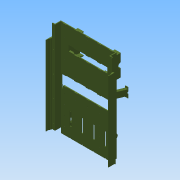
# Autodesk Inventor part: 载板上盖
Saved by Autodesk Inventor 2015 (Build 190159000, 159)
## iProperties
Created: 2017-05-12
Part Number: 载板上盖
Material: 常规
Document SubType Name: Modeling
Designer: Administrator
Density: 1 g/cm^3
Appearance: 橄榄绿
Author: Administrator
Autodesk Inventor part; units mm, degrees
ref_plane "YZ Plane" through (0, 0, 0) normal (1, 0, 0) x (0, 1, 0)
ref_plane "XZ Plane" through (0, 0, 0) normal (0, 1, 0) x (-1, 0, 0)
ref_plane "XY Plane" through (0, 0, 0) normal (0, 0, 1) x (1, 0, 0)
sketch "草图1" plane through (0, 0, 0) normal (0, 0, 1) x (1, 0, 0)
  line L0 (325, 8) -> (325, 0)
  line L1 (325, 0) -> (-325, 0)
  line L2 (-325, 0) -> (-325, 8)
  line L3 (-325, 0) -> (-320, 0)
  line L4 (-320, 0) -> (-320, -52.5)
  line L5 (-320, -52.5) -> (-325, -52.5)
  line L6 (-325, -52.5) -> (-325, 0)
  line L7 (-315, -12.5) -> (-310, -12.5)
  line L8 (-310, -12.5) -> (-310, 0)
  line L9 (325, 0) -> (320, 0)
  line L10 (320, 0) -> (320, -52.5)
  line L11 (320, -52.5) -> (325, -52.5)
  line L12 (325, -52.5) -> (325, 0)
  line L13 (310, 0) -> (310, -12.5)
  line L14 (310, -12.5) -> (315, -12.5)
  line L15 (315, -12.5) -> (315, -22.5)
  line L16 (315, -22.5) -> (320, -27.5)
  line L17 (-315, -12.5) -> (-315, -22.5)
  line L18 (-315, -22.5) -> (-320, -27.5)
  line L19 (-288, 0) -> (-280, 0)
  line L20 (-280, 0) -> (-280, 60)
  line L21 (-280, 60) -> (-288, 60)
  line L22 (-288, 60) -> (-288, 0)
  line L23 (288, 0) -> (280, 0)
  line L24 (280, 0) -> (280, 60)
  line L25 (280, 60) -> (288, 60)
  line L26 (288, 60) -> (288, 0)
  line L27 (-288, 60) -> (288, 60)
  line L28 (288, 60) -> (288, 68)
  line L29 (288, 68) -> (-288, 68)
  line L30 (-288, 68) -> (-288, 60)
  line L31 (-325, 8) -> (-280, 8)
  line L32 (280, 8) -> (325, 8)
  point P0 (0, 0)
  point P1 (0, 0)
  dimension "d0" = 650
  dimension "d1" = 8
  dimension "d2" = 5
  dimension "d3" = 52.5
  dimension "d4" = 12.5
  dimension "d5" = 5
  dimension "d8" = 5
  dimension "d9" = 12.5
  dimension "d10" = 5
  dimension "d11" = 10
  dimension "d12" = 5
  dimension "d14" = 45
  dimension "d15" = 10
  dimension "d16" = 5
  dimension "d17" = 135
  dimension "d18" = 10
  dimension "d19" = 8
  dimension "d20" = 30
  dimension "d21" = 60
  dimension "d22" = 8
  dimension "d23" = 30
  dimension "d24" = 60
  dimension "d25" = 8
  dimension "d26" = 8
  constraints: 66 end point, 14 parallel, 10 perpendicular, 8 point on line, 7 horizontal, 2 vertical, 1 coincident, 1 collinear, 1 midpoint
  measures "d0" distance of L0.end L1.end
  measures "d1" distance of L0.start L0.end
  measures "d2" distance of L4.end L5.end
  measures "d3" distance of L5.end L1.end
  measures "d4" distance of L7.end L8.end
  measures "d5" distance of L7.start L7.end
  measures "d8" distance of L11.end L10.end
  measures "d9" distance of L13.start L13.end
  measures "d10" distance of L13.end L14.end
  measures "d11" distance of L14.end L15.end
  measures "d12" distance from line of L10 L15.end
  measures "d14" angle of L10 L16
  measures "d15" distance of L7.start L17.end
  measures "d16" distance between parallel lines of L4 L17
  measures "d17" angle of L4 L18
  measures "d18" distance between parallel lines of L4 L8
  measures "d19" distance of L21.end L20.end
  measures "d20" distance between parallel lines of L8 L20
  measures "d21" distance of L21.end L19.start
  measures "d22" distance of L24.end L25.end
  measures "d23" distance between parallel lines of L13 L24
  measures "d24" distance of L25.end L23.start
  measures "d25" distance between parallel lines of L27 L29
  measures "d26" distance between parallel lines of L1 L31
extrude "拉伸1" add sketch "草图1" along normal blind 900 contours L0 L1 L26 L32 | L12 L11 L10 L1 | L32 L24 L25 L26 | L26 L1 L24 L32 | L10 L16 L15 L14 L13 L1 | L25 L27 L21 L30 L29 L28 | L20 L31 L22 L21 | L1 L22 L31 L20 | L1 L2 L31 L22 | L8 L7 L17 L18 L4 L1 | L4 L5 L6 L1
sketch "草图2" plane through (-325, -52.5, 0) normal (-1, 0, 0) x (0, 0, 1)
  line L0 (767.5, 60.5) -> (900, 60.5)
  line L1 (900, 60.5) -> (900, 0)
  line L2 (900, 0) -> (767.5, 0)
  line L3 (767.5, 0) -> (767.5, 60.5)
  line L4 (0, 60.5) -> (900, 60.5) projected
  point P0 (0, 52.5)
  dimension "d29" = 132.5
  constraints: 8 end point, 2 parallel, 1 coincident, 1 collinear, 1 horizontal, 1 perpendicular
  measures "d29" distance of L1.end L2.end
extrude "拉伸2" cut sketch "草图2" against normal blind 15
sketch "草图3" plane through (325, -52.5, 0) normal (1, 0, 0) x (0, 0, -1)
  line L0 (-900, 0) -> (-767.5, 0)
  line L1 (-767.5, 0) -> (-767.5, 60.5)
  line L2 (-767.5, 60.5) -> (-900, 60.5)
  line L3 (-900, 60.5) -> (-900, 0)
  line L4 (0, 60.5) -> (-900, 60.5) projected
  point P0 (0, 52.5)
  dimension "d32" = 132.5
  constraints: 8 end point, 2 parallel, 1 collinear, 1 horizontal, 1 perpendicular
  measures "d32" distance of L0.start L0.end
extrude "拉伸3" cut sketch "草图3" against normal blind 15
sketch "草图4" plane through (-325, 8, 0) normal (0, 1, 0) x (1, 0, 0)
  circle A0 centre (26, -10) radius 4
  line L0 (0, 0) -> (0, -767.5) projected
  line L1 (37, 0) -> (0, 0) projected
  circle A1 centre (624, -10) radius 4
  line L2 (650, 0) -> (650, -767.5) projected
  line L3 (650, 0) -> (613, 0) projected
  point P0 (325, 0)
  dimension "d35" = 8
  dimension "d36" = 26
  dimension "d37" = 10
  dimension "d38" = 8
  dimension "d39" = 26
  dimension "d40" = 10
  constraints: 2 centre point
  measures "d35" diameter of A0
  measures "d36" distance from line of L0 A0.centre
  measures "d37" distance from line of L1 A0.centre
  measures "d38" diameter of A1
  measures "d39" distance from line of L2 A1.centre
  measures "d40" distance from line of L3 A1.centre
extrude "拉伸4" cut sketch "草图4" against normal blind 8
pattern_linear "矩形阵列1" count 5 spacing 220 along (0, 0, 1) of "拉伸4"
sketch "草图5" plane through (0, 0, 0) normal (0, 0, -1) x (-1, 0, 0)
  line L0 (-288, 8) -> (-325, 8)
  line L1 (-325, 8) -> (-288, 8) projected
  line L2 (-325, 8) -> (-325, -52.5)
  line L3 (-325, -52.5) -> (-320.7269, -52.5)
  line L4 (-320.7269, -52.5) -> (-320, -52.5)
  line L5 (-320, -27.5) -> (-320, -52.5) projected
  line L6 (-320, -52.5) -> (-320, -27.5)
  line L7 (-320, -27.5) -> (-315, -22.5)
  line L8 (-315, -22.5) -> (-320, -27.5) projected
  line L9 (-315, -22.5) -> (-315, -12.5)
  line L10 (-315, -12.5) -> (-310, -12.5)
  line L11 (-310, -12.5) -> (-315, -12.5) projected
  line L12 (-310, -12.5) -> (-310, 0)
  line L13 (-310, 0) -> (-280, 0)
  line L14 (-280, 0) -> (-280, 60)
  line L15 (-280, 60) -> (280, 60)
  line L16 (280, 60) -> (280, 0)
  line L17 (280, 0) -> (310, 0)
  line L18 (310, 0) -> (280, 0) projected
  line L19 (310, 0) -> (310, -12.5)
  line L20 (310, -12.5) -> (315, -12.5)
  line L21 (315, -12.5) -> (310, -12.5) projected
  line L22 (315, -12.5) -> (315, -22.5)
  line L23 (315, -22.5) -> (315, -12.5) projected
  line L24 (315, -22.5) -> (320, -27.5)
  line L25 (320, -27.5) -> (315, -22.5) projected
  line L26 (320, -27.5) -> (320, -52.5)
  line L27 (320, -52.5) -> (325, -52.5)
  line L28 (325, -52.5) -> (325, 8)
  line L29 (325, 8) -> (288, 8)
  line L30 (288, 8) -> (288, 68)
  line L31 (288, 68) -> (-288, 68)
  line L32 (-288, 68) -> (-288, 8)
  point P0 (0, 0)
  constraints: 50 end point, 15 perpendicular, 8 collinear, 2 parallel, 1 point on line
extrude "拉伸5" add sketch "草图5" along normal blind 50
sketch "草图6" plane through (-288, 68, 900) normal (0, 1, 0) x (1, 0, 0)
  line L0 (89, 172) -> (487, 172)
  line L1 (487, 172) -> (487, 228)
  line L2 (487, 228) -> (89, 228)
  line L3 (89, 228) -> (89, 172)
  line L4 (288, 228) -> (288, 172)
  line L5 (89, 200) -> (487, 200)
  line L6 (576, 0) -> (0, 0) projected
  line L7 (613, 950) -> (613, 132.5) projected
  point P0 (288, 900)
  dimension "d48" = 398
  dimension "d49" = 56
  dimension "d50" = 200
  dimension "d51" = 325
  constraints: 12 end point, 4 midpoint, 2 parallel, 1 horizontal, 1 perpendicular
  measures "d48" distance of L2.end L1.end
  measures "d49" distance of L2.end L0.start
  measures "d50" distance between parallel lines of L6 L5
  measures "d51" distance between parallel lines of L7 L4
extrude "拉伸6" cut sketch "草图6" against normal through all
sketch "草图7" plane through (-288, 68, 900) normal (0, 1, 0) x (1, 0, 0)
  line L0 (526, 460) -> (15, 460)
  line L1 (15, 460) -> (15, 560)
  line L2 (15, 560) -> (526, 560)
  line L3 (526, 560) -> (526, 460)
  line L4 (576, 0) -> (0, 0) projected
  line L5 (0, 950) -> (0, 0) projected
  line L6 (576, 950) -> (576, 0) projected
  point P0 (288, 900)
  dimension "d54" = 460
  dimension "d55" = 560
  dimension "d56" = 15
  dimension "d57" = 50
  constraints: 8 end point, 2 parallel, 1 horizontal, 1 perpendicular
  measures "d54" distance between parallel lines of L4 L0
  measures "d55" distance between parallel lines of L4 L2
  measures "d56" distance between parallel lines of L5 L1
  measures "d57" distance between parallel lines of L6 L3
extrude "拉伸7" cut sketch "草图7" against normal blind 8
sketch "草图8" plane through (-288, 68, 900) normal (0, 1, 0) x (1, 0, 0)
  line L0 (115.5, 892) -> (100.5, 892)
  line L1 (100.5, 892) -> (100.5, 755)
  line L2 (100.5, 755) -> (115.5, 755)
  line L3 (115.5, 755) -> (115.5, 892)
  line L4 (576, 0) -> (0, 0) projected
  line L5 (0, 950) -> (0, 0) projected
  point P0 (288, 900)
  dimension "d60" = 15
  dimension "d61" = 755
  dimension "d62" = 892
  dimension "d63" = 100.5
  constraints: 8 end point, 2 parallel, 1 horizontal, 1 perpendicular
  measures "d60" distance of L1.end L2.end
  measures "d61" distance between parallel lines of L4 L2
  measures "d62" distance between parallel lines of L4 L0
  measures "d63" distance between parallel lines of L5 L1
extrude "拉伸8" cut sketch "草图8" against normal blind 8
pattern_linear "矩形阵列2" count 4 spacing 120 along (1, 0, 0) of "拉伸8"
sketch "草图9" plane through (0, 0, 900) normal (0, 0, 1) x (1, 0, 0)
  line L0 (-273, 60) -> (238, 60) projected
  line L1 (-225, 60) -> (-220, 55)
  line L2 (-220, 55) -> (-260, 55)
  line L3 (-260, 55) -> (-255, 60)
  line L4 (-280, 0) -> (-280, 60) projected
  point P0 (0, 0)
  dimension "d69" = 20
  dimension "d70" = 40
  dimension "d71" = 30
  dimension "d72" = 25
  dimension "d73" = 5
  constraints: 6 end point, 2 point on line, 1 parallel
  measures "d69" distance from line of L4 L2.end
  measures "d70" distance of L2.end L1.end
  measures "d71" distance of L1.start L3.end
  measures "d72" distance from line of L4 L3.end
  measures "d73" distance between parallel lines of L0 L2
extrude "拉伸9" add sketch "草图9" against normal blind 950
pattern_linear "矩形阵列3" count 5 spacing 120 along (1, 0, 0) of "拉伸9"
sketch "草图10" plane through (-288, 68, 900) normal (0, 1, 0) x (1, 0, 0)
  line L0 (526, 560) -> (15, 560)
  line L1 (15, 560) -> (15, 460)
  line L2 (15, 460) -> (526, 460)
  line L3 (487, 228) -> (89, 228)
  line L4 (89, 172) -> (487, 172)
  line L5 (513, 460) -> (513, 560) projected
  line L6 (526, 460) -> (15, 460) projected
  line L7 (15, 560) -> (526, 560) projected
  line L8 (15, 460) -> (15, 560) projected
  line L9 (89, 228) -> (89, 172)
  line L10 (487, 172) -> (89, 172) projected
  line L11 (89, 228) -> (487, 228) projected
  line L12 (487, 228) -> (487, 172)
  line L13 (526, 460) -> (526, 560)
  line L14 (513, 460) -> (526, 460) projected
  point P0 (288, 900)
  constraints: 16 end point, 6 point on line, 5 collinear, 2 horizontal, 2 parallel, 2 perpendicular, 2 vertical
extrude "拉伸10" cut sketch "草图10" against normal blind 13
sketch "草图11" plane through (-260, 55, 900) normal (0, -1, 0) x (1, 0, 0)
  circle A0 centre (20, -25) radius 2.5
  line L0 (0, 0) -> (40, 0) projected
  line L1 (0, 0) -> (0, -460) projected
  point P0 (260, -900)
  dimension "d81" = 5
  dimension "d82" = 25
  dimension "d83" = 20
  constraints: 1 centre point
  measures "d81" diameter of A0
  measures "d82" distance from line of L0 A0.centre
  measures "d83" distance from line of L1 A0.centre
extrude "拉伸11" cut sketch "草图11" against normal blind 13
thread "螺纹1" size "M5x0.8" class "6H" standard "ANSI Metric M Profile" full length
pattern_linear "矩形阵列4" count 5 spacing 100 along (0, 0, -1) of "拉伸11" skipped copies 3
sketch "草图12" plane through (-260, 55, 340) normal (0, -1, 0) x (1, 0, 0)
  circle A0 centre (20, -365) radius 2.5
  line L0 (40, -390) -> (0, -390) projected
  point P0 (260, -340)
  dimension "d91" = 5
  dimension "d92" = 25
  dimension "d93" = 20
  constraints: 1 centre point
  measures "d91" diameter of A0
  measures "d92" distance from line of L0 A0.centre
  measures "d93" horizontal distance of L0.start A0.centre
extrude "拉伸12" cut sketch "草图12" against normal blind 13
thread "螺纹2" size "M5x0.8" class "6H" standard "ANSI Metric M Profile" full length
pattern_linear "矩形阵列5" count 4 spacing 100 along (0, 0, 1) of "拉伸12"
pattern_linear "矩形阵列6" count 5 spacing 120 along (1, 0, 0) of "拉伸11", "矩形阵列4", "拉伸12", "矩形阵列5"
sketch "草图13" plane through (-288, 68, 900) normal (0, 1, 0) x (1, 0, 0)
  line L0 (523, 710) -> (40, 710)
  line L1 (40, 710) -> (40, 690)
  line L2 (40, 690) -> (523, 690)
  line L3 (523, 690) -> (523, 710)
  line L4 (0, 950) -> (0, 0) projected
  line L5 (576, 0) -> (0, 0) projected
  point P0 (288, 900)
  dimension "d104" = 483
  dimension "d105" = 40
  dimension "d106" = 20
  dimension "d107" = 690
  constraints: 8 end point, 2 parallel, 1 horizontal, 1 perpendicular
  measures "d104" distance of L2.end L1.end
  measures "d105" distance between parallel lines of L4 L1
  measures "d106" distance of L0.end L1.end
  measures "d107" distance between parallel lines of L5 L2
extrude "拉伸13" add sketch "草图13" along normal blind 22
fillet "圆角1" radius 10 2 edges at (-6.5, 90, 190) (-6.5, 90, 210)
sketch "草图14" plane through (-248, 68, 190) normal (-1, 0, 0) x (0, 0, 1)
  circle A0 centre (10, 12) radius 5
  arc A1 (20, 12) -> (0, 12) centre (10, 12) ccw projected
  point P0 (-190, -68)
  dimension "d111" = 10
  constraints: 1 centre point, 1 concentric
  measures "d111" diameter of A0
extrude "拉伸14" cut sketch "草图14" against normal through all
sketch "草图15" plane through (-288, 68, 900) normal (0, 1, 0) x (1, 0, 0)
  line L0 (40, 710) -> (523, 710) projected
  line L1 (523, 690) -> (40, 690) projected
  line L2 (100, 710) -> (181, 710)
  line L3 (181, 710) -> (181, 690)
  line L4 (181, 690) -> (100, 690)
  line L5 (100, 690) -> (100, 710)
  line L6 (241, 690) -> (322, 690)
  line L7 (322, 690) -> (322, 710)
  line L8 (322, 710) -> (241, 710)
  line L9 (241, 710) -> (241, 690)
  line L10 (382, 690) -> (463, 690)
  line L11 (463, 690) -> (463, 710)
  line L12 (463, 710) -> (382, 710)
  line L13 (382, 710) -> (382, 690)
  line L14 (40, 690) -> (40, 710) projected
  line L15 (523, 710) -> (523, 690) projected
  point P0 (288, 900)
  dimension "d114" = 81
  dimension "d115" = 81
  dimension "d116" = 81
  dimension "d117" = 60
  dimension "d118" = 60
  dimension "d119" = 60
  constraints: 24 end point, 6 parallel, 6 point on line, 3 horizontal, 3 perpendicular
  measures "d114" distance of L3.end L4.end
  measures "d115" distance of L8.end L7.end
  measures "d116" distance of L12.end L11.end
  measures "d117" distance between parallel lines of L14 L5
  measures "d118" distance from line of L10.end L15
  measures "d119" distance between parallel lines of L7 L13
extrude "拉伸15" cut sketch "草图15" along normal through all contours L0 L3 L1 L5 | L0 L7 L1 L9 | L0 L11 L1 L13
ref_plane "工作平面1" through (-248, 8, 900) normal (-1, 0, 0) x (0, 0, 1)
sketch "草图16" plane through (-248, 8, 900) normal (-1, 0, 0) x (0, 0, 1)
  line L0 (-950, 60) -> (0, 60) projected
  line L1 (-450, 60) -> (-502.3989, 235.379)
  line L2 (-390.5103, 60) -> (-450, 60)
  line L3 (-390.5103, 60) -> (-442.9091, 235.379)
  line L4 (-502.3989, 235.379) -> (-442.9091, 235.379)
  line L5 (0, 60) -> (0, 0) projected
  line L6 (-522.654, 235.379) -> (-422.654, 235.379)
  line L7 (-422.654, 235.379) -> (-422.654, 230.379)
  line L8 (-422.654, 230.379) -> (-522.654, 230.379)
  line L9 (-522.654, 230.379) -> (-522.654, 235.379)
  arc A0 (-483.154, 235.379) -> (-462.154, 235.379) centre (-472.654, 235.379) ccw
  line L10 (-441.4153, 230.379) -> (-442.9091, 235.379)
  line L11 (-422.654, 235.379) -> (-422.654, 230.379)
  line L12 (-502.3989, 235.379) -> (-522.654, 235.379)
  line L13 (-522.654, 230.379) -> (-500.905, 230.379)
  line L14 (-502.3989, 235.379) -> (-500.905, 230.379)
  line L15 (-500.905, 230.379) -> (-522.654, 230.379)
  line L16 (-522.654, 230.379) -> (-522.654, 235.379)
  line L17 (-522.654, 235.379) -> (-502.3989, 235.379)
  point P0 (-900, -8)
  dimension "d123" = 57
  dimension "d124" = 175.379
  dimension "d125" = 450
  dimension "d126" = 472.654
  dimension "d127" = 100
  dimension "d128" = 5
  dimension "d129" = 10.5
  constraints: 32 end point, 8 point on line, 6 collinear, 3 parallel, 2 coincident, 2 horizontal, 2 midpoint, 2 perpendicular, 2 point on circle, 1 centre point, 1 vertical
  measures "d123" distance between parallel lines of L3 L1
  measures "d124" distance between parallel lines of L0 L4
  measures "d125" distance from line of L5 point (-450, 60)
  measures "d126" distance from line of point (-472.654, 235.379) L5
  measures "d127" distance of L7.end L8.end
  measures "d128" distance of L6.end L7.end
  measures "d129" radius of A0
extrude "拉伸16" add sketch "草图16" against normal blind 30 contours L1 L8 A0 L3 L0 | L8 L9 L6 L1 | L1 L4 A0 L8 | L8 A0 L4 L3 | L3 L6 L7 L8
pattern_linear "矩形阵列7" count 2 spacing 453 along (1, 0, 0) of "拉伸16"
sketch "草图17" plane through (-218, 8, 900) normal (1, 0, 0) x (0, 0, -1)
  circle A0 centre (472.654, 235.379) radius 18.5
  arc A1 (462.154, 235.379) -> (483.154, 235.379) centre (472.654, 235.379) ccw projected
  point P0 (900, -8)
  dimension "d135" = 37
  constraints: 1 centre point, 1 concentric
  measures "d135" diameter of A0
extrude "拉伸17" cut sketch "草图17" against normal blind 9
sketch "草图18" plane through (-227, 8, 900) normal (1, 0, 0) x (0, 0, -1)
  circle A0 centre (472.654, 235.379) radius 14
  arc A1 (462.154, 235.379) -> (483.154, 235.379) centre (472.654, 235.379) ccw projected
  point P0 (900, -8)
  dimension "d138" = 28
  constraints: 1 centre point, 1 concentric
  measures "d138" diameter of A0
extrude "拉伸18" cut sketch "草图18" against normal blind 5
sketch "草图19" plane through (205, 243.379, 437.846) normal (-1, 0, 0) x (0, 0, 1)
  circle A0 centre (-10.5, 0) radius 18.5
  arc A1 (-21, 0) -> (0, 0) centre (-10.5, 0) ccw projected
  point P0 (-437.846, -243.379)
  dimension "d141" = 37
  constraints: 1 centre point, 1 concentric
  measures "d141" diameter of A0
extrude "拉伸19" cut sketch "草图19" against normal blind 9
sketch "草图20" plane through (214, 243.379, 437.846) normal (-1, 0, 0) x (0, 0, 1)
  circle A0 centre (-10.5, 0) radius 14
  arc A1 (-21, 0) -> (0, 0) centre (-10.5, 0) ccw projected
  point P0 (-437.846, -243.379)
  dimension "d144" = 28
  constraints: 1 centre point, 1 concentric
  measures "d144" diameter of A0
extrude "拉伸20" cut sketch "草图20" against normal blind 5
fillet "圆角2" radius 4 8 edges at (-233, 238.379, 458.5847) (-233, 238.379, 399.095) (-233, 68, 509.4897) (-233, 68, 450) (220, 68, 450) (220, 68, 509.4897) (220, 238.379, 458.5847) (220, 238.379, 399.095)
sketch "草图21" plane through (-248, 243.379, 477.346) normal (0, 1, 0) x (1, 0, 0)
  circle A0 centre (7, 7) radius 2.5
  circle A1 centre (23, 7) radius 2.5
  circle A2 centre (7, 93) radius 2.5
  circle A3 centre (23, 93) radius 2.5
  line L0 (30, 100) -> (30, 68.5) projected
  line L1 (0, 100) -> (30, 100) projected
  line L2 (0, 100) -> (0, 81.2306) projected
  line L3 (30, 31.5) -> (30, 0) projected
  line L4 (0, 0) -> (30, 0) projected
  line L5 (0, 0) -> (0, 39.5) projected
  point P0 (248, 477.346)
  dimension "d148" = 5
  dimension "d149" = 5
  dimension "d150" = 5
  dimension "d151" = 5
  dimension "d152" = 7
  dimension "d153" = 7
  dimension "d154" = 7
  dimension "d155" = 7
  dimension "d156" = 7
  dimension "d157" = 7
  dimension "d158" = 7
  dimension "d159" = 7
  constraints: 4 centre point
  measures "d148" diameter of A0
  measures "d149" diameter of A1
  measures "d150" diameter of A2
  measures "d151" diameter of A3
  measures "d152" distance from line of L0 A3.centre
  measures "d153" distance from line of A3.centre L1
  measures "d154" distance from line of L1 A2.centre
  measures "d155" distance from line of L2 A2.centre
  measures "d156" distance from line of L3 A1.centre
  measures "d157" distance from line of L4 A1.centre
  measures "d158" distance from line of L4 A0.centre
  measures "d159" distance from line of L5 A0.centre
extrude "拉伸21" cut sketch "草图21" against normal blind 5
pattern_linear "矩形阵列8" count 2 spacing 453 along (1, 0, 0) of "拉伸21"
sketch "草图22" plane through (-248, 8, 900) normal (-1, 0, 0) x (0, 0, 1)
  circle A0 centre (-800, 99.5) radius 25
  line L0 (-821.6506, 112) -> (-851.6728, 60)
  line L1 (-892, 60) -> (-755, 60) projected
  line L2 (-950, 60) -> (0, 60) projected
  line L3 (-748.3272, 60) -> (-778.3494, 112)
  line L4 (-851.6728, 60) -> (-748.3272, 60)
  line L5 (0, 60) -> (0, 0) projected
  point P0 (-900, -8)
  dimension "d165" = 50
  dimension "d166" = 60
  dimension "d167" = 39.5
  dimension "d168" = 800
  constraints: 6 end point, 2 point on circle, 2 point on line, 2 tangent, 1 centre point, 1 collinear, 1 equal length
  measures "d165" diameter of A0
  measures "d166" angle of L2 L3
  measures "d167" distance from line of L1 A0.centre
  measures "d168" distance from line of L5 A0.centre
extrude "拉伸22" add sketch "草图22" against normal blind 18
pattern_linear "矩形阵列9" count 2 spacing 465 along (1, 0, 0) of "拉伸22"
sketch "草图23" plane through (-248, 8, 900) normal (-1, 0, 0) x (0, 0, 1)
  circle A0 centre (-800, 99.5) radius 25
  arc A1 (-778.3494, 112) -> (-821.6506, 112) centre (-800, 99.5) ccw projected
  line L0 (-892, 60) -> (-755, 60) projected
  line L1 (-825, 60) -> (-825, 106.1987)
  line L2 (-851.6728, 60) -> (-821.6506, 112) projected
  line L3 (-775, 60) -> (-775, 106.1987)
  line L4 (-778.3494, 112) -> (-748.3272, 60) projected
  line L5 (-825, 106.1987) -> (-821.6506, 112)
  arc A2 (-778.3494, 112) -> (-821.6506, 112) centre (-800, 99.5) ccw projected
  line L6 (-775, 106.1987) -> (-778.3494, 112)
  line L7 (-825, 60) -> (-775, 60)
  point P0 (-900, -8)
  dimension "d174" = 50
  constraints: 10 end point, 4 point on line, 4 tangent, 1 centre point, 1 collinear, 1 concentric, 1 horizontal, 1 parallel, 1 vertical
  measures "d174" diameter of A0
extrude "拉伸23" cut sketch "草图23" against normal blind 5 contours A0 | L3 L0 L1 A0 | A0 L4 L3 | L1 L2 A0
sketch "草图24" plane through (-243, 8, 900) normal (-1, 0, 0) x (0, 0, 1)
  circle A0 centre (-800, 99.5) radius 16
  arc A1 (-778.3494, 112) -> (-821.6506, 112) centre (-800, 99.5) ccw projected
  point P0 (-900, -8)
  dimension "d177" = 32
  constraints: 1 centre point, 1 concentric
  measures "d177" diameter of A0
extrude "拉伸24" cut sketch "草图24" against normal blind 13
sketch "草图25" plane through (217, 107.5, 100) normal (-1, 0, 0) x (0, 0, 1)
  circle A0 centre (0, 0) radius 16
  arc A1 (21.6506, 12.5) -> (-21.6506, 12.5) centre (0, 0) ccw projected
  point P0 (-100, -107.5)
  dimension "d180" = 32
  constraints: 1 centre point, 1 concentric
  measures "d180" diameter of A0
extrude "拉伸25" cut sketch "草图25" against normal blind 9
sketch "草图26" plane through (226, 107.5, 100) normal (-1, 0, 0) x (0, 0, 1)
  circle A0 centre (0, 0) radius 12
  circle A1 centre (0, 0) radius 16 projected
  point P0 (-100, -107.5)
  dimension "d183" = 24
  constraints: 1 centre point, 1 concentric
  measures "d183" diameter of A0
extrude "拉伸26" cut sketch "草图26" against normal blind 3 contours A0
sketch "草图27" plane through (229, 107.5, 100) normal (-1, 0, 0) x (0, 0, 1)
  circle A0 centre (0, 0) radius 7.5
  circle A1 centre (0, 0) radius 12 projected
  point P0 (-100, -107.5)
  dimension "d186" = 15
  constraints: 1 centre point, 1 concentric
  measures "d186" diameter of A0
extrude "拉伸27" cut sketch "草图27" against normal through all contours A0
sketch "草图28" plane through (-243, 8, 900) normal (-1, 0, 0) x (0, 0, 1)
  circle A0 centre (-815, 70) radius 2
  circle A1 centre (-785, 70) radius 2
  circle A2 centre (-785, 113.4732) radius 2
  circle A3 centre (-815, 113.4732) radius 2
  line L0 (-775, 106.1987) -> (-775, 60) projected
  line L1 (-950, 60) -> (0, 60) projected
  line L2 (-825, 60) -> (-825, 106.1987) projected
  arc A4 (-785, 113.4732) -> (-815, 113.4732) centre (-800, 99.5) ccw
  arc A5 (-778.3494, 112) -> (-821.6506, 112) centre (-800, 99.5) ccw projected
  point P0 (-900, -8)
  dimension "d189" = 4
  dimension "d190" = 4
  dimension "d191" = 4
  dimension "d192" = 4
  dimension "d193" = 10
  dimension "d194" = 10
  dimension "d195" = 10
  dimension "d196" = 10
  dimension "d197" = 20.5
  dimension "d198" = 10
  dimension "d199" = 10
  constraints: 5 centre point, 2 point on circle, 1 concentric
  measures "d189" diameter of A0
  measures "d190" diameter of A1
  measures "d191" diameter of A2
  measures "d192" diameter of A3
  measures "d193" distance from line of A1.centre L0
  measures "d194" distance from line of L1 A1.centre
  measures "d195" distance from line of L1 A0.centre
  measures "d196" distance from line of L2 A0.centre
  measures "d197" radius of A4
  measures "d198" distance from line of L0 A2.centre
  measures "d199" distance from line of L2 A3.centre
extrude "拉伸28" cut sketch "草图28" against normal blind 13
sketch "草图29" plane through (-288, 68, 900) normal (0, 1, 0) x (1, 0, 0)
  line L0 (66, 310) -> (89, 310)
  line L1 (89, 310) -> (89, 90)
  line L2 (89, 90) -> (66, 90)
  line L3 (66, 90) -> (66, 310)
  line L4 (576, 0) -> (0, 0) projected
  line L5 (0, 950) -> (0, 0) projected
  line L6 (487, 310) -> (510, 310)
  line L7 (510, 310) -> (510, 90)
  line L8 (510, 90) -> (487, 90)
  line L9 (487, 90) -> (487, 310)
  line L10 (576, 950) -> (576, 0) projected
  point P0 (288, 900)
  dimension "d202" = 23
  dimension "d203" = 90
  dimension "d204" = 66
  dimension "d205" = 220
  dimension "d206" = 23
  dimension "d207" = 90
  dimension "d208" = 66
  dimension "d209" = 220
  constraints: 16 end point, 4 parallel, 2 horizontal, 2 perpendicular
  measures "d202" distance of L1.end L2.end
  measures "d203" distance between parallel lines of L4 L2
  measures "d204" distance between parallel lines of L5 L3
  measures "d205" distance of L0.end L1.end
  measures "d206" distance of L7.end L8.end
  measures "d207" distance between parallel lines of L4 L8
  measures "d208" distance between parallel lines of L10 L7
  measures "d209" distance of L8.end L6.start
extrude "拉伸29" add sketch "草图29" along normal blind 109.5
sketch "草图30" plane through (-222, 68, 590) normal (-1, 0, 0) x (0, 0, 1)
  circle A0 centre (110, 109.5) radius 26
  line L0 (0, 109.5) -> (220, 109.5) projected
  point P0 (-590, -68)
  point P1 (110, 109.5)
  dimension "d212" = 52
  constraints: 1 centre point, 1 coincident, 1 midpoint
  measures "d212" diameter of A0
extrude "拉伸30" cut sketch "草图30" against normal through all
sketch "草图31" plane through (-222, 68, 590) normal (-1, 0, 0) x (0, 0, 1)
  circle A0 centre (84.3674, 83.8674) radius 2.5
  circle A1 centre (135.6326, 83.8674) radius 2.5
  arc A2 (84.3674, 83.8674) -> (135.6326, 83.8674) centre (110, 109.5) ccw
  arc A3 (84, 109.5) -> (136, 109.5) centre (110, 109.5) ccw projected
  line L0 (135.6326, 83.8674) -> (110, 109.5)
  line L1 (110, 109.5) -> (84.3674, 83.8674)
  line L2 (136, 109.5) -> (220, 109.5) projected
  point P0 (-590, -68)
  dimension "d215" = 5
  dimension "d216" = 5
  dimension "d217" = 36.25
  dimension "d218" = 45
  constraints: 4 end point, 3 centre point, 2 point on circle, 1 concentric, 1 perpendicular
  measures "d215" diameter of A0
  measures "d216" diameter of A1
  measures "d217" radius of A2
  measures "d218" angle of L2 L0
extrude "拉伸31" cut sketch "草图31" against normal through all contours A0 A2 L1 | L1 A2 A0 | A2 L0 A1 | A1 L0 A2
thread "螺纹3" size "M5x0.8" class "6H" standard "ANSI Metric M Profile" full length
thread "螺纹4" size "M5x0.8" class "6H" standard "ANSI Metric M Profile" full length
thread "螺纹5" size "M5x0.8" class "6H" standard "ANSI Metric M Profile" full length
thread "螺纹6" size "M5x0.8" class "6H" standard "ANSI Metric M Profile" full length
sketch "草图32" plane through (199, 60, 672) normal (-1, 0, 0) x (0, 0, 1)
  arc A0 (2, 117.5) -> (54, 117.5) centre (28, 117.5) ccw projected
  line L0 (138, 117.5) -> (54, 117.5) projected
  line L1 (131, 117.5) -> (138, 117.5)
  line L2 (138, 117.5) -> (138, 8)
  line L3 (138, 8) -> (138, 117.5) projected
  line L4 (138, 8) -> (-82, 8)
  line L5 (-82, 8) -> (-82, 117.5)
  line L6 (-82, 8) -> (-82, 117.5) projected
  line L7 (-82, 117.5) -> (-75, 117.5)
  line L8 (2, 117.5) -> (-82, 117.5) projected
  line L9 (0, 18.3789) -> (0, 8)
  line L10 (138, 8) -> (-82, 8) projected
  line L11 (56, 18.3789) -> (56, 8)
  arc A1 (56, 18.3789) -> (131, 117.5) centre (28, 117.5) ccw
  arc A2 (-75, 117.5) -> (0, 18.3789) centre (28, 117.5) ccw
  arc A3 (2, 117.5) -> (54, 117.5) centre (28, 117.5) ccw projected
  point P0 (-672, -60)
  dimension "d230" = 56
  dimension "d231" = 103
  dimension "d232" = 103
  constraints: 14 end point, 4 point on circle, 4 point on line, 3 equal length, 2 centre point, 1 concentric, 1 horizontal, 1 parallel, 1 perpendicular, 1 vertical
  measures "d230" distance between parallel lines of L11 L9
  measures "d231" radius of A2
  measures "d232" radius of A1
extrude "拉伸32" add sketch "草图32" along normal blind 38 contours A2 L9 L4 L5 L7 | L0 L2 L4 L11 A1
pattern_linear "矩形阵列10" count 2 spacing 360 along (-1, 0, 0) of "拉伸32"
sketch "草图33" plane through (-288, 177.5, 900) normal (0, 1, 0) x (1, 0, 0)
  circle A0 centre (498.5, 255) radius 4
  circle A1 centre (498.5, 145) radius 4
  circle A2 centre (77.5, 255) radius 4
  circle A3 centre (77.5, 145) radius 4
  line L0 (510, 90) -> (449, 90) projected
  line L1 (510, 226) -> (510, 310) projected
  line L2 (510, 90) -> (510, 174) projected
  line L3 (66, 90) -> (127, 90) projected
  line L4 (89, 226) -> (89, 303) projected
  line L5 (89, 97) -> (89, 174) projected
  point P0 (288, 900)
  dimension "d238" = 8
  dimension "d239" = 8
  dimension "d240" = 8
  dimension "d241" = 8
  dimension "d242" = 110
  dimension "d243" = 55
  dimension "d244" = 11.5
  dimension "d245" = 11.5
  dimension "d246" = 110
  dimension "d247" = 55
  dimension "d248" = 11.5
  dimension "d249" = 11.5
  constraints: 4 centre point
  measures "d238" diameter of A0
  measures "d239" diameter of A1
  measures "d240" diameter of A2
  measures "d241" diameter of A3
  measures "d242" distance of A1.centre A0.centre
  measures "d243" distance from line of L0 A1.centre
  measures "d244" distance from line of L1 A0.centre
  measures "d245" distance from line of L2 A1.centre
  measures "d246" distance of A3.centre A2.centre
  measures "d247" distance from line of L3 A3.centre
  measures "d248" distance from line of L4 A2.centre
  measures "d249" distance from line of L5 A3.centre
extrude "拉伸33" cut sketch "草图33" against normal blind 22
thread "螺纹7" size "M8x1.25" class "6H" standard "ANSI Metric M Profile" full length
thread "螺纹8" size "M8x1.25" class "6H" standard "ANSI Metric M Profile" full length
thread "螺纹9" size "M8x1.25" class "6H" standard "ANSI Metric M Profile" full length
thread "螺纹10" size "M8x1.25" class "6H" standard "ANSI Metric M Profile" full length
sketch "草图34" plane through (0, 0, -50) normal (0, 0, -1) x (-1, 0, 0)
  line L0 (288, 68) -> (-288, 68) projected
  line L1 (-280, 68) -> (280, 68)
  line L2 (280, 68) -> (280, 60)
  line L3 (280, 60) -> (-280, 60)
  line L4 (-280, 60) -> (-280, 68)
  line L5 (-280, 0) -> (-280, 60) projected
  line L6 (-280, 60) -> (-255, 60) projected
  line L7 (280, 60) -> (280, 0) projected
  point P0 (0, 0)
  constraints: 8 end point, 3 collinear, 2 parallel, 1 horizontal, 1 perpendicular, 1 point on line
extrude "拉伸34" add sketch "草图34" along normal blind 50
sketch "草图35" plane through (-288, 68, 900) normal (0, 1, 0) x (1, 0, 0)
  line L0 (108, 980) -> (113, 1000)
  line L1 (8, 1000) -> (568, 1000) projected
  line L2 (108, 980) -> (103, 1000)
  line L3 (113, 1000) -> (103, 1000)
  line L4 (115.5, 892) -> (115.5, 755) projected
  point P0 (288, 900)
  dimension "d262" = 10
  dimension "d263" = 20
  dimension "d264" = 7.5
  constraints: 6 end point, 2 point on line, 1 collinear, 1 equal length
  measures "d262" distance of L2.end L0.end
  measures "d263" distance from line of L1 L0.start
  measures "d264" distance from line of L4 L0.start
sketch "草图36" plane through (0, 0, -100) normal (0, 0, -1) x (-1, 0, 0)
  line L0 (280, 68) -> (-280, 68) projected
  point P0 (0, 0)
  point P1 (180, 40)
  point P2 (187.5, 68)
  dimension "d265" = 28
  dimension "d266" = 7.5
  measures "d265" distance from line of L0 point (180, 40)
  measures "d266" horizontal distance of point (187.5, 68) point (180, 40)
loft "放样1" cut profiles "草图35" section 1 point at (-180, 40, -100)
sketch "草图37" plane through (-288, 68, 900) normal (0, 1, 0) x (1, 0, 0)
  circle A0 centre (101.3269, 997) radius 1.5
  circle A1 centre (111.1731, 983) radius 1.5
  circle A2 centre (114.6731, 997) radius 1.5
  line L0 (108, 980) -> (103, 1000) projected
  line L1 (113, 1000) -> (568, 1000) projected
  line L2 (118, 1000) -> (98, 1000)
  line L3 (98, 1000) -> (98, 980)
  line L4 (98, 980) -> (118, 980)
  line L5 (118, 980) -> (118, 1000)
  line L6 (98, 1000) -> (103, 980)
  line L7 (118, 1000) -> (113, 980)
  line L8 (113, 1000) -> (108, 980) projected
  circle A3 centre (104.8269, 983) radius 1.5
  point P0 (288, 900)
  dimension "d272" = 3
  dimension "d273" = 3
  dimension "d274" = 3
  dimension "d276" = 20
  dimension "d277" = 2.5
  dimension "d278" = 3
  dimension "d279" = 2.5
  dimension "d280" = 2.5
  dimension "d281" = 2.5
  dimension "d282" = 3
  dimension "d283" = 3
  dimension "d284" = 3
  dimension "d285" = 3
  constraints: 12 end point, 4 centre point, 4 parallel, 3 point on line, 1 horizontal, 1 midpoint, 1 perpendicular
  measures "d272" diameter of A0
  measures "d273" diameter of A1
  measures "d274" diameter of A2
  measures "d276" distance of L3.end L4.end
  measures "d277" distance from line of L6 A0.centre
  measures "d278" diameter of A3
  measures "d279" distance from line of A3.centre L6
  measures "d280" distance from line of A1.centre L7
  measures "d281" distance from line of L7 A2.centre
  measures "d282" distance from line of L4 A3.centre
  measures "d283" distance from line of L4 A1.centre
  measures "d284" distance from line of L2 A2.centre
  measures "d285" distance from line of L2 A0.centre
extrude "拉伸35" cut sketch "草图37" against normal through all contours A0 | A1 | A2 | A3
thread "螺纹11" size "M3x0.5" class "6H" standard "ANSI Metric M Profile" full length
thread "螺纹12" size "M3x0.5" class "6H" standard "ANSI Metric M Profile" full length
thread "螺纹13" size "M3x0.5" class "6H" standard "ANSI Metric M Profile" full length
thread "螺纹14" size "M3x0.5" class "6H" standard "ANSI Metric M Profile" full length
pattern_linear "矩形阵列11" count 4 spacing 120 along (1, 0, 0) of "放样1", "拉伸35"
sketch "草图38" plane through (-248, 8, 900) normal (-1, 0, 0) x (0, 0, 1)
  line L0 (-950, 60) -> (0, 60) projected
  line L1 (-865, 60) -> (-735, 60)
  line L2 (-735, 60) -> (-735, 164.5)
  line L3 (-735, 164.5) -> (-865, 164.5)
  line L4 (-865, 164.5) -> (-865, 60)
  circle A0 centre (-800, 99.5) radius 25
  arc A1 (-778.3494, 112) -> (-821.6506, 112) centre (-800, 99.5) ccw projected
  line L5 (-855, 154.5) -> (-745, 154.5)
  line L6 (-745, 154.5) -> (-745, 144.5)
  line L7 (-745, 144.5) -> (-855, 144.5)
  line L8 (-855, 144.5) -> (-855, 154.5)
  line L9 (-851.6728, 60) -> (-821.6506, 112)
  arc A2 (-778.3494, 112) -> (-821.6506, 112) centre (-800, 99.5) ccw projected
  line L10 (-825, 106.1987) -> (-851.6728, 60) projected
  line L11 (-778.3494, 112) -> (-748.3272, 60)
  point P0 (-900, -8)
  dimension "d299" = 130
  dimension "d300" = 65
  dimension "d301" = 104.5
  dimension "d302" = 10
  dimension "d303" = 10
  dimension "d304" = 10
  dimension "d305" = 10
  constraints: 20 end point, 4 parallel, 3 tangent, 2 horizontal, 2 perpendicular, 2 point on line, 1 centre point, 1 collinear, 1 concentric
  measures "d299" distance of L2.end L3.end
  measures "d300" distance from line of L2 A0.centre
  measures "d301" distance of L1.end L2.end
  measures "d302" distance between parallel lines of L2 L6
  measures "d303" distance between parallel lines of L5 L3
  measures "d304" distance between parallel lines of L4 L8
  measures "d305" distance of L7.end L5.start
extrude "拉伸36" add sketch "草图38" against normal blind 18 contours L4 L3 L2 L0 L11 A0 L9
fillet "圆角3" radius 5 6 edges at (-239, 172.5, 165) (-239, 172.5, 35) (-239, 152.5, 45) (-239, 162.5, 45) (-239, 162.5, 155) (-239, 152.5, 155)
sketch "草图39" plane through (-288, 68, 900) normal (0, 1, 0) x (1, 0, 0)
  line L0 (43, 975) -> (23, 975)
  line L1 (23, 975) -> (23, 925)
  line L2 (23, 925) -> (43, 925)
  line L3 (43, 925) -> (43, 975)
  line L4 (8, 1000) -> (103, 1000) projected
  line L5 (40, 825) -> (40, 865) projected
  point P0 (288, 900)
  dimension "d309" = 25
  dimension "d310" = 3
  dimension "d311" = 20
  dimension "d312" = 50
  constraints: 8 end point, 2 parallel, 1 horizontal, 1 perpendicular
  measures "d309" distance between parallel lines of L4 L0
  measures "d310" distance between parallel lines of L5 L3
  measures "d311" distance of L0.start L0.end
  measures "d312" distance of L0.end L1.end
extrude "拉伸37" add sketch "草图39" along normal blind 114.5
sketch "草图40" plane through (-265, 68, -75) normal (-1, 0, 0) x (0, 0, 1)
  circle A0 centre (25, 89.5) radius 16
  circle A1 centre (25, 89.5) radius 25
  line L0 (50, 0) -> (50, 114.5) projected
  line L1 (0, 114.5) -> (50, 114.5) projected
  point P0 (75, -68)
  dimension "d315" = 32
  dimension "d316" = 50
  constraints: 2 centre point, 2 tangent, 1 coincident
  measures "d315" diameter of A0
  measures "d316" diameter of A1
extrude "拉伸38" cut sketch "草图40" against normal blind 20 contours A0
fillet "圆角4" radius 25 2 edges at (-255, 182.5, -75) (-255, 182.5, -25)
sketch "草图41" plane through (-310, 8, 900) normal (0, 1, 0) x (1, 0, 0)
  line L0 (-15, 950) -> (-15, 132.5) projected
  line L1 (-15, 440) -> (22, 440)
  line L2 (22, 440) -> (22, 400)
  line L3 (22, 400) -> (-15, 400)
  line L4 (-15, 400) -> (-15, 440)
  line L5 (22, 0) -> (0, 0) projected
  point P0 (310, 900)
  dimension "d320" = 37
  dimension "d321" = 40
  dimension "d322" = 400
  constraints: 8 end point, 2 parallel, 1 horizontal, 1 perpendicular, 1 point on line
  measures "d320" distance of L2.end L3.end
  measures "d321" distance of L1.end L2.end
  measures "d322" distance between parallel lines of L5 L3
extrude "拉伸39" add sketch "草图41" along normal blind 160
sketch "草图42" plane through (-325, 8, 500) normal (0, 0, 1) x (1, 0, 0)
  line L0 (37, 160) -> (27, 160)
  line L1 (27, 160) -> (27, 60)
  line L2 (27, 60) -> (37, 60)
  line L3 (37, 60) -> (37, 160)
  line L4 (613, 60) -> (37, 60) projected
  point P0 (325, -8)
  dimension "d325" = 10
  constraints: 8 end point, 2 parallel, 1 collinear, 1 horizontal, 1 perpendicular
  measures "d325" distance of L2.end L1.end
extrude "拉伸40" cut sketch "草图42" against normal through all
sketch "草图44" plane through (-265, 68, -75) normal (-1, 0, 0) x (0, 0, 1)
  circle A0 centre (24.984, 31.848) radius 7.5
  line L0 (-25, -8) -> (-25, 0) projected
  line L1 (25, 0) -> (-25, 0) projected
  point P0 (75, -68)
  dimension "d332" = 15
  dimension "d333" = 49.984
  dimension "d334" = 31.848
  constraints: 1 centre point
  measures "d332" diameter of A0
  measures "d333" distance from line of L0 A0.centre
  measures "d334" distance from line of A0.centre L1
extrude "拉伸42" add sketch "草图44" along normal blind 31.27
sketch "草图45" plane through (-296.27, 99.848, -50.016) normal (-1, 0, 0) x (0, 0, 1)
  circle A0 centre (0, 0) radius 10
  circle A1 centre (0, 0) radius 7.5 projected
  point P0 (50.016, -99.848)
  dimension "d337" = 20
  constraints: 1 centre point, 1 concentric
  measures "d337" diameter of A0
extrude "拉伸43" add sketch "草图45" along normal blind 2 contours A0 | A1
sketch "草图46" plane through (-325, -52.5, 767.5) normal (-1, 0, 0) x (0, 0, 1)
  circle A0 centre (-286.993, 194.931) radius 16
  line L0 (-307.5, 60.5) -> (-307.5, 220.5) projected
  line L1 (-267.5, 120.5) -> (132.5, 120.5) projected
  point P0 (-767.5, 52.5)
  dimension "d340" = 32
  dimension "d341" = 20.507
  dimension "d342" = 74.431
  constraints: 1 centre point
  measures "d340" diameter of A0
  measures "d341" distance from line of L0 A0.centre
  measures "d342" distance from line of L1 A0.centre
extrude "拉伸44" cut sketch "草图46" against normal up to surface (27 mm away)
sketch "草图47" plane through (-325, -52.5, 767.5) normal (-1, 0, 0) x (0, 0, 1)
  line L0 (-312.562, 220.5) -> (-261.424, 220.5)
  line L1 (-261.424, 220.5) -> (-261.424, 169.362)
  line L2 (-261.424, 169.362) -> (-312.562, 169.362)
  line L3 (-312.562, 169.362) -> (-312.562, 220.5)
  circle A0 centre (-286.993, 194.931) radius 25.569
  circle A1 centre (-286.993, 194.931) radius 16 projected
  line L4 (-307.5, 220.5) -> (-267.5, 220.5) projected
  circle A2 centre (-286.993, 194.931) radius 16
  point P0 (-767.5, 52.5)
  dimension "d345" = 32
  constraints: 8 end point, 4 tangent, 2 centre point, 2 parallel, 1 coincident, 1 collinear, 1 concentric, 1 horizontal, 1 perpendicular
  measures "d345" diameter of A2
extrude "拉伸45" add sketch "草图47" against normal up to surface (27 mm away)
fillet "圆角6" radius 5 4 edges at (-311.5, 168, 506.076) (-311.5, 116.862, 506.076) (-311.5, 168, 454.938) (-311.5, 116.862, 454.938)
sketch "草图48" plane through (-325, -52.5, 767.5) normal (-1, 0, 0) x (0, 0, 1)
  circle A0 centre (-286.399, 96.714) radius 7.5
  line L0 (-307.5, 60.5) -> (-307.5, 169.362) projected
  line L1 (-267.5, 120.5) -> (132.5, 120.5) projected
  point P0 (-767.5, 52.5)
  dimension "d349" = 15
  dimension "d350" = 21.101
  dimension "d351" = 23.786
  constraints: 1 centre point
  measures "d349" diameter of A0
  measures "d350" distance from line of L0 A0.centre
  measures "d351" distance from line of L1 A0.centre
extrude "拉伸46" add sketch "草图48" along normal blind 26.27
sketch "草图49" plane through (-351.27, 44.214, 481.101) normal (-1, 0, 0) x (0, 0, 1)
  circle A0 centre (0, 0) radius 10
  circle A1 centre (0, 0) radius 7.5 projected
  point P0 (-481.101, -44.214)
  dimension "d354" = 20
  constraints: 1 centre point, 1 concentric
  measures "d354" diameter of A0
extrude "拉伸47" add sketch "草图49" along normal blind 2 contours A0 | A1
sketch "草图50" plane through (-288, 68, 900) normal (0, 1, 0) x (1, 0, 0)
  line L0 (36, 586) -> (19, 586)
  line L1 (19, 586) -> (19, 560)
  line L2 (19, 560) -> (36, 560)
  line L3 (36, 560) -> (36, 586)
  line L4 (0, 950) -> (0, 440) projected
  line L5 (15, 560) -> (526, 560) projected
  point P0 (288, 900)
  dimension "d357" = 26
  dimension "d358" = 17
  dimension "d359" = 19
  constraints: 8 end point, 2 parallel, 1 collinear, 1 horizontal, 1 perpendicular
  measures "d357" distance of L2.end L0.start
  measures "d358" distance of L0.start L0.end
  measures "d359" distance between parallel lines of L4 L1
extrude "拉伸48" cut sketch "草图50" against normal through all
